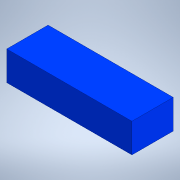
# Autodesk Inventor part: turnigy_battery
Saved by Autodesk Inventor 2020.4 (Build 244396000, 396)
## iProperties
Created: 2021-05-29
Part Number: turnigy_battery
Material: Generic
Document SubType Name: Modeling
Designer: Tarsoly
Density: 1 g/cm^3
Appearance: Default
Author: Tarsoly
Autodesk Inventor part; units mm, degrees
ref_plane "YZ Plane" through (0, 0, 0) normal (1, 0, 0) x (0, 1, 0)
ref_plane "XZ Plane" through (0, 0, 0) normal (0, 1, 0) x (-1, 0, 0)
ref_plane "XY Plane" through (0, 0, 0) normal (0, 0, 1) x (1, 0, 0)
sketch "Sketch1" plane through (0, 0, 0) normal (0, 1, 0) x (-1, 0, 0)
  line L0 (51.5, 17) -> (-51.5, 17)
  line L1 (-51.5, 17) -> (-51.5, -17)
  line L2 (-51.5, -17) -> (51.5, -17)
  line L3 (51.5, -17) -> (51.5, 17)
  line L4 (51.5, 17) -> (-51.5, -17) construction
  line L5 (-51.5, 17) -> (51.5, -17) construction
  point P0 (0, 0)
  dimension "d0" = 103
  dimension "d1" = 34
  constraints: 12 end point, 2 midpoint, 2 parallel, 1 horizontal, 1 perpendicular
  measures "d0" distance of L1.end L2.end
  measures "d1" distance of L2.end L0.start
extrude "Extrusion1" add sketch "Sketch1" along normal blind 24
body "Solid1"
